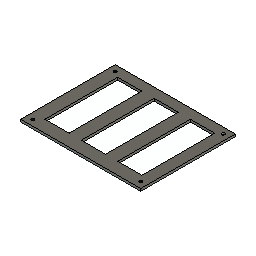
ttop (Autodesk Fusion 360 design; units mm, degrees)
part number: 2026-02-02-21-21-02-304
Autodesk Fusion 360 part; units mm, degrees
sketch "Boceto1" plane through (0, 0, 0) normal (0, 0, 1) x (1, 0, 0)
  line L0 (0, 0) -> (99, 0)
  line L1 (99, 0) -> (99, 78)
  line L2 (99, 78) -> (0, 78)
  line L3 (0, 78) -> (0, 0)
  dimension "d1" = 99
  dimension "d2" = 78
  constraint horizontal L0
  constraint vertical L1
  constraint horizontal L2
  constraint vertical L3
  constraint coincident L0.start L3.end
  measures "d1" distance of L0.start L0.end
  measures "d2" distance of L0.start L2.end
extrude "Extruir1" add sketch "Boceto1" along normal blind 2
sketch "Boceto2" plane through (0, 0, 0) normal (0, 0, -1) x (1, 0, 0)
  line L0 (0, 0) -> (0, -78)
  line L1 (0, -78) -> (99, -78)
  line L2 (99, -78) -> (99, 0)
  line L3 (99, 0) -> (0, 0)
  line L4 (5, -5) -> (5, 0) construction
  constraint coincident L3 L4.end
  constraint perpendicular L3 L4
hole "Agujero1" at (5, 5, 0) direction (0, 0, 1) diameter 5.2 depth 1.2 tip angle 118
sketch "Boceto3" plane through (0, 0, 0) normal (0, 0, -1) x (1, 0, 0)
  circle A0 centre (5, -5) radius 2.6
  line L0 (0, 0) -> (0, -78)
  line L1 (0, -78) -> (99, -78)
  line L2 (99, -78) -> (99, 0)
  line L3 (99, 0) -> (0, 0)
ref_plane "PlanoDeObra3" through (49.5, 39, 1) normal (0, 1, 0) x (-1, 0, 0)
sketch "Boceto4" plane through (0, 0, 0) normal (0, 0, -1) x (1, 0, 0)
  line L0 (5, -73) -> (0, -73) construction
  line L1 (94, -73) -> (94, -78) construction
  line L2 (94, 0) -> (94, -5) construction
  constraint horizontal L0
  constraint vertical L1
  constraint vertical L2
hole "Agujero2" at (94, 5, 0) at (94, 73, 0) at (5, 73, 0) direction (0, 0, 1) diameter 5.2 depth 1.2 tip angle 118
sketch "Boceto5" plane through (0, 0, 2) normal (0, 0, 1) x (-1, 0, 0)
  circle A0 centre (-94, -73) radius 1.2686
  circle A1 centre (-94, -5) radius 1.2686
  circle A2 centre (-5, -73) radius 1.2686
  circle A3 centre (-5, -5) radius 1.2686
  line L0 (0, -78) -> (0, 0)
  line L1 (0, 0) -> (-99, 0)
  line L2 (-99, 0) -> (-99, -78)
  line L3 (-99, -78) -> (0, -78)
  line L4 (-10, -70) -> (-29.8878, -70)
  line L5 (-29.8878, -70) -> (-29.8878, -10)
  line L6 (-29.8878, -10) -> (-10, -10)
  line L7 (-10, -10) -> (-10, -70)
  line L8 (-90, -70) -> (-70.001, -70)
  line L9 (-70.001, -70) -> (-70.001, -10)
  line L10 (-70.001, -10) -> (-90, -10)
  line L11 (-90, -10) -> (-90, -70)
  line L12 (-40, -70) -> (-60, -70)
  line L13 (-60, -70) -> (-60, -10)
  line L14 (-60, -10) -> (-40, -10)
  line L15 (-40, -10) -> (-40, -70)
  constraint horizontal L4
  constraint vertical L5
  constraint horizontal L6
  constraint vertical L7
  constraint horizontal L8
  constraint vertical L9
  constraint horizontal L10
  constraint vertical L11
  constraint horizontal L12
  constraint vertical L13
  constraint horizontal L14
  constraint vertical L15
extrude "Extruir2" cut sketch "Boceto5" against normal blind 5 contours L4 L5 L6 L7 | L8 L9 L10 L11 | L12 L13 L14 L15
equation "d10 = ( -78 / 2 ) * 1 mm"
